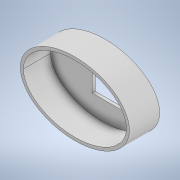
# Autodesk Inventor part: fleet2
Saved by Autodesk Inventor 2020 (Build 240168000, 168)
## iProperties
Created: 2020-01-04
Part Number: fleet2
Material: Generic
Document SubType Name: Modeling
Designer: my
Density: 1 g/cm^3
Appearance: Default
Author: my
Autodesk Inventor part; units mm, degrees
ref_plane "YZ Plane" through (0, 0, 0) normal (1, 0, 0) x (0, 1, 0)
ref_plane "XZ Plane" through (0, 0, 0) normal (0, 1, 0) x (-1, 0, 0)
ref_plane "XY Plane" through (0, 0, 0) normal (0, 0, 1) x (1, 0, 0)
sketch "Sketch1" plane through (0, 0, 0) normal (0, 0, 1) x (1, 0, 0)
  ellipse E0 centre (0, 0) end of major axis (90, 0) minor radius 60
  dimension "d2" = 60
  dimension "d3" = 90
  constraints: 1 centre point, 1 other
extrude "Extrusion1" add sketch "Sketch1" along normal blind 50
shell "Shell1" thickness 5 removed faces 1 at (-2.0197, -19.8984, 50)
sketch "Sketch2" plane through (5.8562, 2.0528, 5) normal (0, 0, 1) x (1, 0, 0)
  line L0 (-22.3219, -24.5537) -> (27.6781, -24.5537)
  line L1 (27.6781, -24.5537) -> (27.6781, 25.4463)
  line L2 (27.6781, 25.4463) -> (-22.3219, 25.4463)
  line L3 (-22.3219, 25.4463) -> (-22.3219, -24.5537)
  line L4 (-22.3219, -24.5537) -> (27.6781, 25.4463) construction
  line L5 (27.6781, -24.5537) -> (-22.3219, 25.4463) construction
  point P0 (-5.8562, -2.0528)
  point P1 (2.6781, 0.4463)
  dimension "d7" = 50
  dimension "d8" = 50
  constraints: 12 end point, 2 midpoint, 2 parallel, 1 horizontal, 1 perpendicular
  measures "d7" distance of L2.end L0.start
  measures "d8" distance of L1.end L2.end
extrude "Extrusion2" cut sketch "Sketch2" against normal blind 10
body "Solid1"
